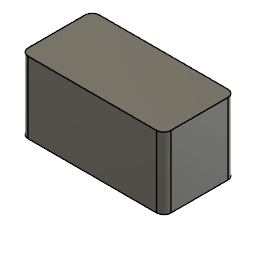
Bottom of box (Autodesk Fusion 360 design; units mm, degrees)
Autodesk Fusion 360 part; units mm, degrees
sketch "Sketch1" plane through (0, 0, 0) normal (0, 1, 0) x (1, 0, 0) in component "Bottom of Box"
  line L0 (-184.0142, 60) -> (15.9858, 60)
  line L1 (15.9858, 60) -> (15.9858, -40)
  line L2 (15.9858, -40) -> (-184.0142, -40)
  line L3 (-184.0142, -40) -> (-184.0142, 60)
  line L4 (-169.0142, 45) -> (0.9858, 45)
  line L5 (0.9858, 45) -> (0.9858, -25)
  line L6 (0.9858, -25) -> (-169.0142, -25)
  line L7 (-169.0142, -25) -> (-169.0142, 45)
  dimension "d1" = 100
  dimension "d2" = 200
  dimension "d3" = 170
  dimension "d4" = 70
  dimension "d5" = 15
  dimension "d6" = 15
  constraint horizontal L0
  constraint vertical L1
  constraint horizontal L2
  constraint vertical L3
  constraint horizontal L4
  constraint vertical L5
  constraint horizontal L6
  constraint vertical L7
  measures "d1" distance of L0 L2
  measures "d2" distance of L1 L3
  measures "d3" distance of L5 L7
  measures "d4" distance of L4 L6
  measures "d5" distance of L0 L4
  measures "d6" distance of L1 L5
extrude "Extrude1" add sketch "Sketch1" along normal blind 100 contours L0 L1 L2 L3 | L4 L5 L6 L7 in component "Bottom of Box"
extrude "Extrude2" cut sketch "Sketch1" along normal blind 85 contours L4 L5 L6 L7 in component "Bottom of Box"
fillet "Fillet1" radius 10 1 edges at (15.9858, 50, -60) in component "Bottom of Box"
fillet "Fillet2" radius 10 1 edges at (15.9858, 50, 40) in component "Bottom of Box"
fillet "Fillet3" radius 10 1 edges at (-184.0142, 50, 40) in component "Bottom of Box"
fillet "Fillet4" radius 10 1 edges at (-184.0142, 50, -60) in component "Bottom of Box"
sketch "Sketch1 (2)" plane through (0, 0, 0) normal (0, 1, 0) x (1, 0, 0)
  line L0 (-69.0142, -25) -> (-99.0142, -25)
  line L1 (-99.0142, -25) -> (-99.0142, 22)
  line L2 (-99.0142, 22) -> (-69.0142, 22)
  line L3 (-69.0142, 22) -> (-69.0142, -25)
  line L4 (0.9858, -25) -> (0.9858, 45)
  dimension "d30" = 30
  dimension "d31" = 70
  dimension "d79" = 47
  constraint horizontal L0
  constraint vertical L1
  constraint horizontal L2
  constraint vertical L3
  measures "d30" distance of L1 L3
  measures "d31" distance of L3 L4
  measures "d79" distance of L0 L2
extrude "Extrude4" add sketch "Sketch1 (2)" along normal blind 20 in component "Bottom of Box"
sketch "Sketch2" plane through (0, 0, 0) normal (0, 1, 0) x (1, 0, 0)
  circle A0 centre (-84.0142, 7) radius 7.5
  line L0 (-99.0142, 22) -> (-69.0142, 22)
  line L1 (-99.0142, -25) -> (-99.0142, 22)
  dimension "d34" = 15
  dimension "d35" = 15
  dimension "d36" = 15
  measures "d34" diameter of A0
  measures "d35" distance of A0.centre L0
  measures "d36" distance of A0.centre L1
extrude "Extrude5" add sketch "Sketch2" against normal blind 25 in component "Bottom of Box"
sketch "Sketch3" plane through (0, 0, 0) normal (1, 0, 0) x (0, 0, -1)
  circle A0 through (-3.7834, -13.0013, 0.7579) (-12.7129, -6.8816, 0.7341) (-13.5467, -17.6734, 0.5639)
  line L0 (-0.5, -25) -> (14.5, -25)
  dimension "d40" = 12.5
  dimension "d81" = 12.5
extrude "Extrude7" cut 1 faces at (-82.4555, -25, -8.9546) along direction (0, 1, 0) blind 10 in component "Bottom of Box"
extrude "Extrude8" add 1 faces at (-82.4555, -15, -8.9546) along direction (0, -1, 0) blind 19 in component "Bottom of Box"
sketch "Sketch5" plane through (0, 0, 0) normal (0, -1, 0) x (1, 0, 0)
  circle A0 centre (-84.0142, -7) radius 7.5
  line L0 (-169.0142, -45) -> (-169.0142, 25)
  line L1 (-169.0142, 25) -> (-99.0142, 25)
  line L2 (-99.0142, 25) -> (-99.0142, -22)
  line L3 (-99.0142, -22) -> (-69.0142, -22)
  line L4 (-69.0142, -22) -> (-69.0142, 25)
  line L5 (-69.0142, 25) -> (0.9858, 25)
  line L6 (0.9858, 25) -> (0.9858, -45)
  line L7 (0.9858, -45) -> (-169.0142, -45)
  arc A1 (-184.0142, -50) -> (-174.0142, -60) centre (-174.0142, -50) ccw
  line L8 (-174.0142, -60) -> (5.9858, -60)
  arc A2 (5.9858, -60) -> (15.9858, -50) centre (5.9858, -50) ccw
  line L9 (15.9858, -50) -> (15.9858, 30)
  arc A3 (15.9858, 30) -> (5.9858, 40) centre (5.9858, 30) ccw
  line L10 (5.9858, 40) -> (-174.0142, 40)
  arc A4 (-174.0142, 40) -> (-184.0142, 30) centre (-174.0142, 30) ccw
  line L11 (-184.0142, 30) -> (-184.0142, -50)
  line L12 (-170.0142, -56) -> (1.9858, -56)
  line L13 (11.9858, -46) -> (11.9858, 26)
  line L14 (1.9858, 36) -> (-170.0142, 36)
  line L15 (-180.0142, 26) -> (-180.0142, -46)
  line L16 (-173.0142, -49) -> (4.9858, -49)
  line L17 (4.9858, -49) -> (4.9858, 29)
  line L18 (4.9858, 29) -> (-173.0142, 29)
  line L19 (-173.0142, 29) -> (-173.0142, -49)
  arc A5 (11.9858, 26) -> (1.9858, 36) centre (1.9858, 26) ccw
  arc A6 (1.9858, -56) -> (11.9858, -46) centre (1.9858, -46) ccw
  arc A7 (-180.0142, -46) -> (-170.0142, -56) centre (-170.0142, -46) ccw
  arc A8 (-170.0142, 36) -> (-180.0142, 26) centre (-170.0142, 26) ccw
  point P0 (-180.0142, -56)
  point P1 (11.9858, -56)
  dimension "d52" = 192
  dimension "d53" = 92
  dimension "d54" = 4
  dimension "d55" = 4
  dimension "d56" = 78
  dimension "d57" = 178
  dimension "d58" = 7
  dimension "d59" = 7
  dimension "d60" = 10
  constraint horizontal L12
  constraint vertical L13
  constraint horizontal L14
  constraint vertical L15
  constraint horizontal L16
  constraint vertical L17
  constraint horizontal L18
  constraint vertical L19
  constraint tangent L13 A5
  constraint tangent L14 A5
  constraint coincident P1 L12
  constraint coincident P1 L13
  constraint tangent L12 A6
  constraint tangent L13 A6
  constraint equal A5 A6
  constraint coincident P0 L12
  constraint coincident P0 L15
  constraint tangent L12 A7
  constraint tangent L15 A7
  constraint equal A5 A7
  constraint tangent L14 A8
  constraint tangent L15 A8
  constraint equal A5 A8
  measures "d52" distance of P0 P1
  measures "d53" distance of L12 L14
  measures "d54" distance of L8 L12
  measures "d55" distance of L9 L13
  measures "d56" distance of L16.end L17.end
  measures "d57" distance of L17 L19
  measures "d58" distance of L15 L19
  measures "d59" distance of L14 L18
  measures "d60" radius of A5
extrude "Extrude10" cut sketch "Sketch5" against normal blind 15 contours L12 L13 L14 L15 A5 A6 A7 A8 in component "Bottom of Box"
sketch "Sketch6" plane through (0, 0, 0) normal (1, 0, 0) x (0, 0, -1)
sketch "Sketch7" plane through (0, 0, 0) normal (1, 0, 0) x (0, 0, -1)
  circle A0 centre (7, -21) radius 5.75
  line L0 (-0.5, -34) -> (14.5, -34)
  dimension "d69" = 7.5
  dimension "d82" = 11.5
  dimension "d84" = 13
  measures "d69" horizontal distance of A0.centre L0.end
  measures "d82" diameter of A0
  measures "d84" distance of A0.centre L0
extrude "Extrude11" cut sketch "Sketch7" against normal blind 100 in component "Bottom of Box"
component "Bottom of Box" placed x (1, 0, 0) y (0, 1, 0) z (0, 0, 1) at (0, 0, 0)
